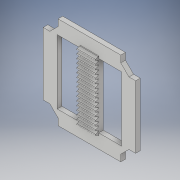
# Autodesk Inventor part: 20_Cube_Insert_focusing_rail_v3
Saved by Autodesk Inventor 2019 (Build 230136000, 136)
## iProperties
Created: 2021-04-22
Part Number: 20_Cube_Insert_focusing_rail_v3
Material: Generic
Document SubType Name: Modeling
Designer: UC2
Density: 1 g/cm^3
Appearance: Default
Author: UC2
Autodesk Inventor part; units mm, degrees
ref_plane "YZ Plane" through (0, 0, 0) normal (1, 0, 0) x (0, 1, 0)
ref_plane "XZ Plane" through (0, 0, 0) normal (0, 1, 0) x (-1, 0, 0)
ref_plane "XY Plane" through (0, 0, 0) normal (0, 0, 1) x (1, 0, 0)
sketch "Skizze4" plane through (0, 0, 0) normal (0, 0, 1) x (1, 0, 0)
  line L0 (-38.36, 0) -> (55.8314, 0) construction
  line L1 (0, -35.8777) -> (0, 40.9376) construction
  line L2 (0, 0) -> (29.964, 29.964) construction
  line L3 (0, 0) -> (42.3755, 0) construction
  line L4 (0, 24.9041) -> (16.9, 24.9041)
  line L5 (16.9, 24.9041) -> (16.9, 21.2841)
  line L6 (16.9, 21.2841) -> (19.092, 19.092)
  line L7 (24.9041, 0) -> (24.9041, 16.9)
  line L8 (24.9041, 16.9) -> (21.2841, 16.9)
  line L9 (21.2841, 16.9) -> (19.092, 19.092)
  line L10 (0, 24.9041) -> (-16.9, 24.9041)
  line L11 (-16.9, 24.9041) -> (-16.9, 21.2841)
  line L12 (-16.9, 21.2841) -> (-19.092, 19.092)
  line L13 (-24.9041, 0) -> (-24.9041, 16.9)
  line L14 (-24.9041, 16.9) -> (-21.2841, 16.9)
  line L15 (-21.2841, 16.9) -> (-19.092, 19.092)
  line L16 (0, -24.9041) -> (16.9, -24.9041)
  line L17 (16.9, -24.9041) -> (16.9, -21.2841)
  line L18 (16.9, -21.2841) -> (19.092, -19.092)
  line L19 (24.9041, 0) -> (24.9041, -16.9)
  line L20 (24.9041, -16.9) -> (21.2841, -16.9)
  line L21 (21.2841, -16.9) -> (19.092, -19.092)
  line L22 (0, -24.9041) -> (-16.9, -24.9041)
  line L23 (-16.9, -24.9041) -> (-16.9, -21.2841)
  line L24 (-16.9, -21.2841) -> (-19.092, -19.092)
  line L25 (-24.9041, 0) -> (-24.9041, -16.9)
  line L26 (-24.9041, -16.9) -> (-21.2841, -16.9)
  line L27 (-21.2841, -16.9) -> (-19.092, -19.092)
  line L28 (-17.3243, 17.3243) -> (-5, 17.3243)
  line L29 (-5, 17.3243) -> (-5, -17.3243)
  line L30 (-5, -17.3243) -> (-17.3243, -17.3243)
  line L31 (-17.3243, -17.3243) -> (-17.3243, 17.3243)
  line L32 (17.3243, 17.3243) -> (5, 17.3243)
  line L33 (5, 17.3243) -> (5, -17.3243)
  line L34 (5, -17.3243) -> (17.3243, -17.3243)
  line L35 (17.3243, -17.3243) -> (17.3243, 17.3243)
  dimension "d17" = 45
  dimension "d18" = 16.9
  dimension "d19" = 3.1
  dimension "d20" = 3.62
  dimension "d21" = 10
  dimension "d22" = 2.5
  constraints: 68 end point, 24 symmetric about line, 3 horizontal, 3 perpendicular, 3 point on line, 2 parallel, 1 equal length, 1 other
  measures "d17" angle of L3 L2
  measures "d18" distance of L4.start L4.end
  measures "d19" distance of L5.end L6.end
  measures "d20" distance of L4.end L5.end
  measures "d21" distance between parallel lines of L29 L33
  measures "d22" distance of L6.end L35.end
extrude "Extrusion2" add sketch "Skizze4" along normal blind 2.5
sketch "Skizze6" plane through (5, -17.3243, 0) normal (1, 0, 0) x (0, 0, -1)
  line L0 (0, 34.6485) -> (0, 0) construction
  line L1 (0, 34.6485) -> (-2.5, 34.6485) construction
  line L2 (-2.5, 0) -> (-2.5, 34.6485) construction
  line L3 (0, 0) -> (-2.5, 0) construction
  line L4 (0, 42.2283) -> (0, 38.6083) construction
  line L5 (0, 42.2283) -> (-2.5, 42.2283) construction
  line L6 (-2.5, 38.6083) -> (-2.5, 42.2283) construction
  line L7 (0, 38.6083) -> (-2.5, 38.6083) construction
  line L8 (0, -3.9598) -> (0, -7.5798) construction
  line L9 (0, -3.9598) -> (-2.5, -3.9598) construction
  line L10 (-2.5, -7.5798) -> (-2.5, -3.9598) construction
  line L11 (0, -7.5798) -> (-2.5, -7.5798) construction
  line L12 (0, 0.4243) -> (0, -3.9598) construction
  line L13 (0, 0.4243) -> (-2.5, 0.4243) construction
  line L14 (-2.5, -3.9598) -> (-2.5, 0.4243) construction
  line L15 (0, -3.9598) -> (-2.5, -3.9598) construction
  line L16 (0, 38.6083) -> (0, 34.2243) construction
  line L17 (0, 38.6083) -> (-2.5, 38.6083) construction
  line L18 (-2.5, 34.2243) -> (-2.5, 38.6083) construction
  line L19 (0, 34.2243) -> (-2.5, 34.2243) construction
  line L20 (0, 34.2243) -> (0, 0.4243) construction
  line L21 (0, 34.2243) -> (-2.5, 34.2243) construction
  line L22 (-2.5, 0.4243) -> (-2.5, 34.2243) construction
  line L23 (0, 0.4243) -> (-2.5, 0.4243) construction
  line L24 (0, 17.3243) -> (-7.845, 17.3243) construction
  line L25 (-2.5, 34.2243) -> (-2.5, 0.4243) projected
  line L26 (-2.5, 18.2083) -> (-4.3794, 17.5243)
  line L27 (-4.3794, 17.5243) -> (-4.3794, 17.1243)
  line L28 (-4.3794, 17.1243) -> (-2.5, 16.4402)
  line L29 (-2.5, 18.2083) -> (-2.5, 16.4402)
  dimension "d25" = 70
  dimension "d26" = 2
  dimension "d27" = 0.4
  constraints: 10 end point, 2 point on line, 1 collinear, 1 horizontal, 1 parallel, 1 other
  measures "d25" angle of L2 L26
  measures "d26" distance of L26.start L26.end
  measures "d27" distance of L26.end L27.end
extrude "Extrusion3" add sketch "Skizze6" against normal up to surface (10 mm away)
fillet "Rundung1" radius 0.3 4 edges at (0, 0.2, 4.3794) (0, -0.2, 4.3794) (0, 0.884, 2.5) (0, -0.884, 2.5)
pattern_linear "Rechteckige Anordnung1" count 17 spacing 2.186 along (0, -1, 0) of "Extrusion3", "Rundung1" first direction both ways yes
